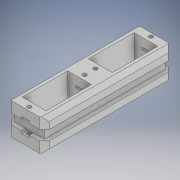
# Autodesk Inventor part: FEMUR2_A
Saved by Autodesk Inventor 2017 (Build 210142000, 142)
## iProperties
Created: 2017-09-24
Part Number: FEMUR2_A
Material: Generic
Document SubType Name: Modeling
Designer: Alexander Miller
Density: 1 g/cm^3
Appearance: Default
Author: Alexander Miller
Autodesk Inventor part; units mm, degrees
ref_plane "YZ Plane" through (0, 0, 0) normal (1, 0, 0) x (0, 1, 0)
ref_plane "XZ Plane" through (0, 0, 0) normal (0, 1, 0) x (-1, 0, 0)
ref_plane "XY Plane" through (0, 0, 0) normal (0, 0, 1) x (1, 0, 0)
sketch "Sketch1" plane through (0, 0, 0) normal (0, 1, 0) x (-1, 0, 0)
  line L0 (32.5, -9.5) -> (-32.5, -9.5)
  line L1 (-32.5, -9.5) -> (-32.5, 9.5)
  line L2 (-32.5, 9.5) -> (32.5, 9.5)
  line L3 (32.5, 9.5) -> (32.5, -9.5)
  point P0 (0, 0)
  point P1 (0, -9.5)
  point P2 (32.5, 0)
  dimension "d0" = 65
  dimension "d1" = 19
  constraints: 8 end point, 2 midpoint, 2 parallel, 1 horizontal, 1 horizontal alignment, 1 perpendicular, 1 vertical alignment
  measures "d0" distance of L0.start L0.end
  measures "d1" distance of L2.end L0.start
extrude "Extrusion1" add sketch "Sketch1" along normal blind 16
sketch "Sketch2" plane through (0, 16, 0) normal (0, 1, 0) x (1, 0, 0)
  line L0 (-28.25, 6) -> (-5.25, 6)
  line L1 (-5.25, 6) -> (-5.25, -6)
  line L2 (-5.25, -6) -> (-28.25, -6)
  line L3 (-28.25, -6) -> (-28.25, 6)
  line L4 (0, 13.3) -> (0, -13.3) construction
  line L5 (-32.5, 9.5) -> (-32.5, -9.5) projected
  line L6 (28.25, 6) -> (5.25, 6)
  line L7 (5.25, 6) -> (5.25, -6)
  line L8 (5.25, -6) -> (28.25, -6)
  line L9 (28.25, -6) -> (28.25, 6)
  point P0 (0, 0)
  point P1 (-5.25, 0)
  dimension "d4" = 23
  dimension "d5" = 12
  dimension "d9" = 4.25
  constraints: 16 end point, 4 symmetric about line, 2 parallel, 1 horizontal, 1 horizontal alignment, 1 midpoint, 1 perpendicular
  measures "d4" distance of L0.start L0.end
  measures "d5" distance of L2.end L0.start
  measures "d9" distance between parallel lines of L5 L3
extrude "Extrusion2" cut sketch "Sketch2" against normal through all
chamfer "Chamfer1" distance 2.5 angle 45 4 edges at (-32.5, 8, 9.5) (-32.5, 8, -9.5) (32.5, 8, 9.5) (32.5, 8, -9.5)
chamfer "Chamfer2" distance 2 angle 45 4 edges at (0, 16, -9.5) (0, 16, 9.5) (0, 0, 9.5) (0, 0, -9.5)
sketch "Sketch3" plane through (-30, 2, 9.5) normal (0, 0, 1) x (1, 0, 0)
  line L0 (-2.5, 8.5) -> (62.5, 8.5)
  line L1 (62.5, 8.5) -> (62.5, 3.5)
  line L2 (62.5, 3.5) -> (-2.5, 3.5)
  line L3 (-2.5, 3.5) -> (-2.5, 8.5)
  line L4 (-2.5, 14) -> (-2.5, -2) projected
  line L5 (62.5, -2) -> (62.5, 14) projected
  point P0 (30, -2)
  point P1 (62.5, 6)
  point P2 (62.5, 6)
  dimension "d18" = 5
  constraints: 8 end point, 2 collinear, 2 midpoint, 2 parallel, 1 coincident, 1 horizontal, 1 perpendicular
  measures "d18" distance between parallel lines of L2 L0
extrude "Extrusion3" cut sketch "Sketch3" against normal blind 2
sketch "Sketch5" plane through (30, 2, -9.5) normal (0, 0, -1) x (-1, 0, 0)
  line L0 (-2.5, 3.5) -> (62.5, 3.5)
  line L1 (62.5, 3.5) -> (62.5, 8.5)
  line L2 (62.5, 8.5) -> (-2.5, 8.5)
  line L3 (-2.5, 8.5) -> (-2.5, 3.5)
  line L4 (-2.5, 14) -> (-2.5, -2) projected
  line L5 (62.5, -2) -> (62.5, 14) projected
  point P0 (30, -2)
  point P1 (62.5, 6)
  point P2 (62.5, 6)
  dimension "d21" = 5
  constraints: 8 end point, 2 collinear, 2 midpoint, 2 parallel, 1 coincident, 1 horizontal, 1 perpendicular
  measures "d21" distance between parallel lines of L0 L2
extrude "Extrusion4" cut sketch "Sketch5" against normal blind 2
sketch "Sketch6" plane through (-32.5, 0, -7) normal (-1, 0, 0) x (0, 0, 1)
  line L0 (-0.5, 5.5) -> (-2.5, 5.5) projected
  line L1 (16.5, 10.5) -> (-2.5, 10.5)
  line L2 (-2.5, 10.5) -> (-2.5, 5.5)
  line L3 (-2.5, 5.5) -> (16.5, 5.5)
  line L4 (16.5, 5.5) -> (16.5, 10.5)
  point P0 (7, 0)
  point P1 (16.5, 5.5)
  point P2 (-2.5, 10.5)
  constraints: 8 end point, 2 parallel, 1 horizontal, 1 perpendicular
extrude "Extrusion5" cut sketch "Sketch6" against normal blind 2
sketch "Sketch7" plane through (32.5, 0, 7) normal (1, 0, 0) x (0, 0, -1)
  line L0 (0, 10.5) -> (-2.5, 10.5) projected
  line L1 (-2.5, 10.5) -> (16.5, 10.5)
  line L2 (16.5, 10.5) -> (16.5, 5.5)
  line L3 (16.5, 5.5) -> (-2.5, 5.5)
  line L4 (-2.5, 5.5) -> (-2.5, 10.5)
  point P0 (7, 0)
  constraints: 8 end point, 2 parallel, 1 horizontal, 1 perpendicular
extrude "Extrusion6" cut sketch "Sketch7" against normal blind 2
sketch "Sketch8" plane through (32.5, 16, 7) normal (1, 0, 0) x (0, 0, -1)
  line L0 (5, -4.3) -> (9, -4.3)
  line L1 (9, -4.3) -> (9, -5.5)
  line L2 (9, -5.5) -> (5, -5.5)
  line L3 (5, -5.5) -> (5, -4.3)
  line L4 (5, -10.5) -> (9, -10.5)
  line L5 (9, -10.5) -> (9, -11.7)
  line L6 (9, -11.7) -> (5, -11.7)
  line L7 (5, -11.7) -> (5, -10.5)
  line L8 (14, -16) -> (0, -16) projected
  line L9 (0, -5.5) -> (14, -5.5) projected
  line L10 (14, -10.5) -> (0, -10.5) projected
  point P0 (7, -16)
  point P1 (7, -4.3)
  point P2 (7, -10.5)
  point P3 (7, -11.7)
  point P4 (7, -16)
  dimension "d28" = 4
  dimension "d29" = 1.2
  constraints: 16 end point, 4 midpoint, 4 parallel, 2 collinear, 2 equal length, 2 horizontal, 2 perpendicular, 2 vertical alignment
  measures "d28" distance of L0.start L0.end
  measures "d29" distance of L2.end L0.start
extrude "Extrusion7" cut sketch "Sketch8" against normal through all
sketch "Sketch9" plane through (0, 16, 0) normal (0, 1, 0) x (1, 0, 0)
  circle A0 centre (30.75, 0) radius 1
  circle A1 centre (2.75, 0) radius 1
  line L0 (0, 13.3) -> (0, -13.3) projected
  line L1 (28.25, 6) -> (28.25, -6) projected
  line L2 (5.25, -6) -> (5.25, 6) projected
  circle A2 centre (-30.75, 0) radius 1
  circle A3 centre (-2.75, 0) radius 1
  point P0 (0, 0)
  dimension "d32" = 2
  dimension "d33" = 1.5
  dimension "d34" = 1.5
  constraints: 4 centre point, 2 horizontal alignment, 2 symmetric about line, 1 equal radius, 2 other
  measures "d32" diameter of A0
  measures "d33" distance edge to line of A0 L1
  measures "d34" distance edge to line of A1 L2
extrude "Extrusion8" cut sketch "Sketch9" against normal up to surface (4.3 mm away)
sketch "Sketch10" plane through (0, 0, 0) normal (0, -1, 0) x (1, 0, 0)
  line L0 (0, -13.3) -> (0, 13.3) projected
  circle A0 centre (-30.75, 0) radius 1
  circle A1 centre (-2.75, 0) radius 1
  line L1 (-28.25, -6) -> (-28.25, 6) projected
  line L2 (-5.25, 6) -> (-5.25, -6) projected
  circle A2 centre (30.75, 0) radius 1
  circle A3 centre (2.75, 0) radius 1
  point P0 (0, 0)
  dimension "d37" = 2
  dimension "d38" = 1.5
  dimension "d39" = 1.5
  constraints: 4 centre point, 2 horizontal alignment, 2 symmetric about line, 1 equal radius, 2 other
  measures "d37" diameter of A0
  measures "d38" distance edge to line of A0 L1
  measures "d39" distance edge to line of A1 L2
extrude "Extrusion9" cut sketch "Sketch10" against normal up to surface (4.3 mm away)
equation "\"d4\" = servo_A"
equation "\"d5\" = servo_B"
equation "\"d9\" = -0.5 * servo_A + 0.5 * servo_D"
equation "\"d18\" = servo_K"
equation "\"d21\" = servo_K"
equation "\"d28\" = nut_A"
equation "\"d29\" = nut_B"
equation "\"d32\" = servo_H"
equation "\"d33\" = servo_L"
equation "\"d34\" = servo_L"
equation "\"d37\" = servo_H"
equation "\"d38\" = servo_L"
equation "\"d39\" = servo_L"
equation "\"servo_A\" = 23"
equation "\"servo_B\" = 12"
equation "\"servo_D\" = 31.5"
equation "\"servo_K\" = 5"
equation "\"nut_A\" = 4"
equation "\"nut_B\" = 1.2"
equation "\"servo_H\" = 2"
equation "\"servo_L\" = 1.5"
body "Solid1"
